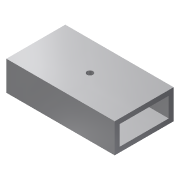
# Autodesk Inventor part: AluminumBlock
Saved by Autodesk Inventor 2014 (Build 180170000, 170)
## iProperties
Created: 2014-08-10
Part Number: AluminumBlock
Material: Generic
Document SubType Name: Modeling
Designer: Peele
Density: 1 g/cm^3
Appearance: Aluminum - Polished
Author: Peele
Autodesk Inventor part; units mm, degrees
ref_plane "YZ Plane" through (0, 0, 0) normal (1, 0, 0) x (0, 1, 0)
ref_plane "XZ Plane" through (0, 0, 0) normal (0, 1, 0) x (-1, 0, 0)
ref_plane "XY Plane" through (0, 0, 0) normal (0, 0, 1) x (1, 0, 0)
sketch "Sketch1" plane through (0, 0, 0) normal (1, 0, 0) x (0, 1, 0)
  line L0 (-15.875, -6.35) -> (15.875, -6.35)
  line L1 (15.875, -6.35) -> (15.875, 6.35)
  line L2 (15.875, 6.35) -> (-15.875, 6.35)
  line L3 (-15.875, 6.35) -> (-15.875, -6.35)
  line L4 (-15.875, -6.35) -> (15.875, 6.35) construction
  line L5 (15.875, -6.35) -> (-15.875, 6.35) construction
  line L6 (-19.05, -9.525) -> (19.05, -9.525)
  line L7 (19.05, -9.525) -> (19.05, 9.525)
  line L8 (19.05, 9.525) -> (-19.05, 9.525)
  line L9 (-19.05, 9.525) -> (-19.05, -9.525)
  line L10 (-19.05, -9.525) -> (19.05, 9.525) construction
  line L11 (19.05, -9.525) -> (-19.05, 9.525) construction
  point P0 (0, 0)
  dimension "d0" = 38.1
  dimension "d1" = 19.05
  dimension "d2" = 3.175
  dimension "d3" = 3.175
  constraints: 24 end point, 4 midpoint, 4 parallel, 2 horizontal, 2 perpendicular
  measures "d0" distance of L6.start L6.end
  measures "d1" distance of L8.end L6.start
  measures "d2" distance between parallel lines of L8 L2
  measures "d3" distance between parallel lines of L9 L3
extrude "Extrusion1" add sketch "Sketch1" along normal mid plane 70
sketch "Sketch2" plane through (-35, -19.05, 9.525) normal (0, 0, 1) x (1, 0, 0)
  circle A0 centre (35, 19.05) radius 2
  dimension "d6" = 4
  constraints: 1 centre point, 1 coincident
  measures "d6" diameter of A0
extrude "Extrusion2" cut sketch "Sketch2" against normal blind 10
equation "\"d3\" = d2"
body "Solid1"
